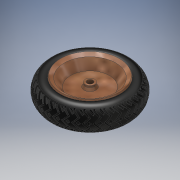
# Autodesk Inventor part: tyre-st3
Saved by Autodesk Inventor 2017 (Build 210142000, 142)
## iProperties
Created: 2017-04-23
Part Number: tyre-st3
Material: Generic
Document SubType Name: Modeling
Designer: master
Density: 1 g/cm^3
Appearance: Glossy - Black
Author: master
Autodesk Inventor part; units mm, degrees
ref_plane "YZ Plane" through (0, 0, 0) normal (1, 0, 0) x (0, 1, 0)
ref_plane "XY Plane" through (0, 0, 0) normal (0, 0, 1) x (1, 0, 0)
sketch "Sketch1" plane through (0, 0, 0) normal (1, 0, 0) x (0, 1, 0)
  arc A0 (19.4611, -0.0269) -> (17.3271, 4.699) centre (13.1611, -0.0269) ccw
  line L0 (1.8558, 0.28) -> (1.8558, 3.1705)
  arc A1 (17.3271, 4.699) -> (13.3967, 4.7312) centre (15.3433, 2.4486) ccw
  line L1 (14.0586, 5.1596) -> (13.7467, 5.6996)
  line L2 (13.7467, 5.6996) -> (12.1337, 4.7679)
  line L3 (9.3395, 1.2421) -> (3.2435, 1.2421)
  line L4 (1.8558, 3.1705) -> (2.6607, 3.1705)
  line L5 (2.6607, 3.1705) -> (2.6607, 2.3756)
  line L6 (2.6607, 2.3756) -> (3.2435, 1.2421)
  line L7 (9.3395, 1.2421) -> (12.1337, 4.7679)
  line L8 (0.5558, -7.3073) -> (0.5558, 7.8674)
  line L9 (13.7467, -5.7534) -> (12.1337, -4.8217)
  line L10 (14.0586, -5.2134) -> (13.7467, -5.7534)
  arc A2 (13.3967, -4.785) -> (17.3271, -4.7528) centre (15.3433, -2.5023) ccw
  line L11 (9.3395, -1.2958) -> (12.1337, -4.8217)
  line L12 (9.3395, -1.2958) -> (3.2435, -1.2958)
  line L13 (2.6607, -2.4294) -> (3.2435, -1.2958)
  line L14 (2.6607, -3.2243) -> (2.6607, -2.4294)
  line L15 (1.8558, -3.2243) -> (2.6607, -3.2243)
  line L16 (1.8558, 0.28) -> (1.8558, -3.2243)
  arc A3 (17.3271, -4.7528) -> (19.4611, -0.0269) centre (13.1611, -0.0269) ccw
  point P0 (0, 0)
  dimension "d0" = 6.3
  dimension "d1" = 128.397
  dimension "d2" = 158.41
  dimension "d3" = 6.096
  dimension "d4" = 1.3
  dimension "d5" = 3
  dimension "d6" = 0.54
  constraints: 34 end point, 14 point on circle, 4 centre point, 2 horizontal, 2 perpendicular, 1 tangent, 1 vertical
  measures "d0" radius of A0
  measures "d1" angle of L7 L3
  measures "d2" angle of L2 L7
  measures "d3" distance of L3.start L3.end
  measures "d4" distance between parallel lines of L8 L16
  measures "d5" radius of A1
  measures "d6" vertical distance of L1.start L2.start
revolve "Revolution1" add sketch "Sketch1" angle 360 about axis through (0, 0.5558, -7.3073) along (0, 0, 1)
ref_plane "Work Plane1" through (0, 19.5, 0) normal (0, 1, 0) x (-1, 0, 0)
sketch "Sketch2" plane through (0, 19.5, 0) normal (0, 1, 0) x (-1, 0, 0)
  line L0 (0, 0) -> (2.056, 2.056)
  line L1 (2.056, 2.056) -> (0, 4.112)
  line L2 (0, 4.112) -> (0.4443, 4.5563)
  line L3 (1.2414, 4.5563) -> (0.7971, 4.112)
  line L4 (0.7971, 4.112) -> (2.8532, 2.056)
  line L5 (2.8532, 2.056) -> (0.7971, 0)
  line L6 (0, 0) -> (2.056, -2.056)
  line L7 (2.056, -2.056) -> (0, -4.112)
  line L8 (1.2414, -4.5563) -> (0.7971, -4.112)
  line L9 (0.7971, -4.112) -> (2.8532, -2.056)
  line L10 (2.8532, -2.056) -> (0.7971, 0)
  line L11 (0, -4.112) -> (0.4443, -4.5563)
  line L12 (1.2414, 4.5563) -> (0.4443, 4.5563)
  line L13 (0.4443, -4.5563) -> (1.2414, -4.5563)
  line L14 (2.056, 4.112) -> (3.4826, 2.6854)
  line L15 (3.4826, 2.6854) -> (3.9843, 3.1872)
  line L16 (3.9843, 3.1872) -> (2.5577, 4.6137)
  line L17 (2.5577, 4.6137) -> (2.056, 4.112)
  line L18 (2.3069, 0.8624) -> (1.4982, 0.0538)
  line L19 (1.4982, 0.0538) -> (2.311, -0.7591)
  line L20 (2.311, -0.7591) -> (3.1197, 0.0496)
  line L21 (3.1197, 0.0496) -> (2.3069, 0.8624)
  line L22 (2.056, -4.112) -> (3.4826, -2.6854)
  line L23 (3.4826, -2.6854) -> (3.9843, -3.1872)
  line L24 (3.9843, -3.1872) -> (2.5577, -4.6137)
  line L25 (2.5577, -4.6137) -> (2.056, -4.112)
  point P0 (5.001, -5.001)
  point P1 (0.2174, 0.2174)
  constraints: 52 end point, 5 parallel, 4 perpendicular
extrude "Extrusion1" cut sketch "Sketch2" against normal blind 3
pattern_circular "Circular Pattern1" count 33 over 360 about axis through (0, 0, -10) along (0, 0, 1) of "Extrusion1"
body "Solid1"
